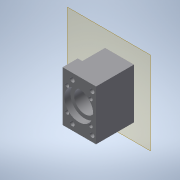
# Autodesk Inventor part: 30_Cube_Z_Focus_NEMA8_captive_motorbase_v0
Saved by Autodesk Inventor 2022 (Build 260153000, 153)
## iProperties
Created: 2022-05-23
Part Number: 30_Cube_Z_Focus_NEMA8_captive_motorbase_v0
Material: Generisch
Document SubType Name: Modeling
Designer: diederichbenedict
Density: 1 g/cm^3
Appearance: Vorgabe
Author: diederichbenedict
Autodesk Inventor part; units mm, degrees
ref_plane "YZ Plane" through (0, 0, 0) normal (1, 0, 0) x (0, 1, 0)
ref_plane "XZ Plane" through (0, 0, 0) normal (0, 1, 0) x (-1, 0, 0)
ref_plane "XY Plane" through (0, 0, 0) normal (0, 0, 1) x (1, 0, 0)
ref_plane "Arbeitsebene1" through (-0.0002, 0, 0) normal (0, 0, 1) x (1, 0, 0)
sketch "Skizze1" plane through (-0.0002, 0, 0) normal (0, 0, 1) x (1, 0, 0)
  circle A0 centre (13.85, 6.86) radius 1.5 projected
  circle A1 centre (0.85, 31.86) radius 1.5 projected
  circle A2 centre (13.85, 31.86) radius 1.5 projected
  circle A3 centre (0.85, 6.86) radius 1.5 projected
  circle A4 centre (5.0933, 19.36) radius 5.5 projected
  line L0 (-3.07, 5.49) -> (-3.07, 33.23) projected
  line L1 (-3.07, 5.49) -> (-16.87, 5.49) projected
  line L2 (-16.87, 13.31) -> (-16.87, 5.49) projected
  line L3 (-16.8476, 13.31) -> (-16.87, 13.31) projected
  line L4 (-16.8476, 25.41) -> (-16.8476, 13.31) projected
  line L5 (-16.87, 25.41) -> (-16.8476, 25.41) projected
  line L6 (-16.87, 33.23) -> (-16.87, 25.41) projected
  line L7 (-3.07, 33.23) -> (-16.87, 33.23) projected
  line L8 (-16.87, 40.13) -> (-16.87, 44.21) projected
  line L9 (-20.77, 36.23) -> (-16.87, 40.13) projected
  line L10 (-24.85, 36.23) -> (-20.77, 36.23) projected
  line L11 (-24.85, 2.49) -> (-24.85, 36.23) projected
  line L12 (-20.77, 2.49) -> (-24.85, 2.49) projected
  line L13 (-16.87, -1.41) -> (-20.77, 2.49) projected
  line L14 (-16.87, -1.41) -> (-16.87, -5.49) projected
  line L15 (-16.87, -5.49) -> (16.87, -5.49) projected
  line L16 (16.87, -5.49) -> (16.87, -1.41) projected
  line L17 (20.77, 2.49) -> (16.87, -1.41) projected
  line L18 (24.85, 2.49) -> (20.77, 2.49) projected
  line L19 (24.85, 36.23) -> (24.85, 2.49) projected
  line L20 (20.77, 36.23) -> (24.85, 36.23) projected
  line L21 (16.87, 40.13) -> (20.77, 36.23) projected
  line L22 (16.87, 44.21) -> (16.87, 40.13) projected
  line L23 (-16.87, 44.21) -> (16.87, 44.21) projected
  line L24 (16.97, 36.33) -> (16.97, 2.39) projected
  line L25 (-16.97, 36.33) -> (16.97, 36.33) construction
  line L26 (-16.97, 2.39) -> (-16.97, 36.33) projected
  line L27 (16.97, 2.39) -> (-16.97, 2.39) construction
  line L28 (16.97, 2.39) -> (-16.97, 2.39) projected
  line L29 (16.47, 35.83) -> (16.47, 2.89)
  line L30 (16.47, 2.89) -> (-16.47, 2.89)
  line L31 (-16.47, 2.89) -> (-16.47, 35.83)
  line L32 (-16.47, 35.83) -> (16.47, 35.83)
  line L33 (-2.57, 35.83) -> (-2.57, 2.89)
  circle A5 centre (5.0933, 19.36) radius 7
  point P0 (0.0002, 0)
  dimension "d0" = 0.5
  dimension "d1" = 0.5
  dimension "d18" = 14
  constraints: 10 end point, 2 point on line, 1 centre point, 1 coincident, 1 parallel, 3 other
  measures "d0" distance between parallel lines of L25 L32
  measures "d1" distance between parallel lines of L0 L33
  measures "d18" diameter of A5
extrude "Extrusion1" add sketch "Skizze1" along normal blind 25 contours L33 L32 L29 L30
sketch "Skizze2" plane through (-2.5702, 2.89, 0) normal (0, -1, 0) x (1, 0, 0)
  line L0 (0, 0) -> (0, 25) projected
  line L1 (0, 25) -> (-3, 25)
  line L2 (-3, 25) -> (-3, 15)
  line L3 (-3, 15) -> (0, 15)
  line L4 (0, 15) -> (0, 25)
  point P0 (2.5702, 0)
  point P1 (0, 15)
  dimension "d4" = 3
  dimension "d5" = 10
  constraints: 8 end point, 2 parallel, 1 horizontal, 1 perpendicular
  measures "d4" distance of L3.end L2.end
  measures "d5" distance of L2.end L1.end
extrude "Extrusion2" add sketch "Skizze2" against normal up to surface (32.94 mm away)
sketch "Skizze3" plane through (-0.0002, 0, 0) normal (0, 0, -1) x (-1, 0, 0)
  circle A0 centre (2.4634, 11.66) radius 1 projected
  circle A1 centre (-13.85, 6.86) radius 1.5 projected
  circle A2 centre (-12.9366, 27.06) radius 1 projected
  circle A3 centre (2.4634, 27.06) radius 1 projected
  circle A4 centre (-12.9366, 27.06) radius 1 projected
  arc A5 (-14.6686, 11.41) -> (-13.1866, 9.9279) centre (-12.9366, 11.66) ccw projected
  arc A6 (-13.1866, 13.3921) -> (-14.6686, 11.91) centre (-12.9366, 11.66) ccw projected
  point P0 (-0.0002, 0)
hole "Bohrung1" at (-2.4636, 11.66, 0) at (-2.4636, 27.06, 0) at (12.9364, 27.06, 0) at (12.9364, 11.66, 0) direction (0, 0, 1) diameter 2.5 end through all counterbore diameter 5 counterbore depth 18
sketch "Skizze4" plane through (-0.0002, 0, 25) normal (0, 0, 1) x (1, 0, 0)
  circle A0 centre (5.0933, 19.36) radius 5.5 projected
  circle A1 centre (5.0933, 19.36) radius 9.5
  point P0 (0.0002, 0)
  dimension "d15" = 19
  constraints: 1 centre point, 1 coincident
  measures "d15" diameter of A1
extrude "Extrusion3" cut sketch "Skizze4" against normal blind 4 contours A0 | A1
